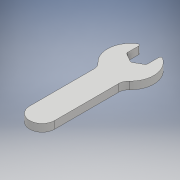
# Autodesk Inventor part: M2ナットレンチ
Saved by Autodesk Inventor 2017 (Build 210142000, 142)
## iProperties
Part Number: M2ナットレンチ
Material: 一般
Document SubType Name: Modeling
Designer: NN
Density: 1 g/cm^3
Appearance: 既定
Author: NN
Autodesk Inventor part; units mm, degrees
ref_plane "YZ Plane" through (0, 0, 0) normal (1, 0, 0) x (0, 1, 0)
ref_plane "XZ Plane" through (0, 0, 0) normal (0, 1, 0) x (-1, 0, 0)
ref_plane "XY Plane" through (0, 0, 0) normal (0, 0, 1) x (1, 0, 0)
sketch "スケッチ1" plane through (0, 0, 0) normal (0, 0, 1) x (1, 0, 0)
  line L0 (0, 2.3094) -> (2, 1.1547)
  line L1 (2, 1.1547) -> (2, -1.1547)
  line L2 (2, -1.1547) -> (0, -2.3094)
  line L3 (0, -2.3094) -> (-2, -1.1547)
  line L4 (-2, -1.1547) -> (-2, 1.1547)
  line L5 (-2, 1.1547) -> (0, 2.3094)
  circle A0 centre (0, 0) radius 3.5
  line L6 (0, 0) -> (0, -20)
  circle A1 centre (0, -20) radius 2.5
  line L7 (2.5, -20) -> (2.5, -2.4495)
  line L8 (-2.5, -20) -> (-2.5, -2.4495)
  line L9 (-2, 1.1547) -> (-3.4875, 0.2959)
  line L10 (2, 1.1547) -> (3.4875, 0.2959)
  circle A2 centre (0, -2.3094) radius 4.6188
  line L11 (2, 1.1547) -> (2, 1.8539)
  line L12 (-2, 1.1547) -> (-2, 1.8539)
  dimension "d0" = 4
  dimension "d1" = 7
  dimension "d2" = 20
  dimension "d3" = 5
  constraints: 26 end point, 9 point on circle, 4 coincident, 4 vertical, 3 centre point, 2 collinear, 2 parallel, 2 tangent, 13 other
  measures "d0" distance between parallel lines of L1 L4
  measures "d1" diameter of A0
  measures "d2" distance of L6.start L6.end
  measures "d3" diameter of A1
extrude "押し出し1" add sketch "スケッチ1" along normal blind 1.5 contours L10 A0 L6 L2 L1 | L11 A2 A0 L10 | L4 L3 L6 A0 L9 | L9 A0 A2 L12 | A0 A2 L7 | A0 L8 A2 | A0 L6 A2 L8 | A2 L6 A1 L8 | A0 L7 A2 L6 | L7 A1 L6 A2 | A1
fillet "フィレット1" radius 0.3 2 edges at (-2, 1.8539, 0.75) (2, 1.8539, 0.75)
fillet "フィレット2" radius 0.5 3 edges at (2, -1.1547, 0.75) (0, -2.3094, 0.75) (-2, -1.1547, 0.75)
fillet "フィレット3" radius 2 2 edges at (-2.5, -6.1931, 0.75) (2.5, -6.1931, 0.75)
